Autodesk Inventor part; units mm, degrees
(part 2 of 2)
sketch "Sketch34" plane through (-87.5594, 7.4535, 25) normal (0, 1, 0) x (1, 0, 0)
  line L0 (67.0332, 20.1615) -> (71.3633, 20.1615)
  line L1 (71.3633, 20.1615) -> (73.5284, 16.4115)
  line L2 (73.5284, 16.4115) -> (71.3633, 12.6615)
  line L3 (71.3633, 12.6615) -> (67.0332, 12.6615)
  line L4 (67.0332, 12.6615) -> (64.8681, 16.4115)
  line L5 (64.8681, 16.4115) -> (67.0332, 20.1615)
  line L6 (76.0332, 14.75) -> (80.3633, 14.75)
  line L7 (80.3633, 14.75) -> (82.5284, 11)
  line L8 (82.5284, 11) -> (80.3633, 7.25)
  line L9 (80.3633, 7.25) -> (76.0332, 7.25)
  line L10 (76.0332, 7.25) -> (73.8681, 11)
  line L11 (73.8681, 11) -> (76.0332, 14.75)
  line L12 (67.0332, 30.9846) -> (71.3633, 30.9846)
  line L13 (71.3633, 30.9846) -> (73.5284, 27.2346)
  line L14 (73.5284, 27.2346) -> (71.3633, 23.4846)
  line L15 (71.3633, 23.4846) -> (67.0332, 23.4846)
  line L16 (67.0332, 23.4846) -> (64.8681, 27.2346)
  line L17 (64.8681, 27.2346) -> (67.0332, 30.9846)
  line L18 (76.0332, 25.5731) -> (80.3633, 25.5731)
  line L19 (80.3633, 25.5731) -> (82.5284, 21.8231)
  line L20 (82.5284, 21.8231) -> (80.3633, 18.0731)
  line L21 (80.3633, 18.0731) -> (76.0332, 18.0731)
  line L22 (76.0332, 18.0731) -> (73.8681, 21.8231)
  line L23 (73.8681, 21.8231) -> (76.0332, 25.5731)
  line L24 (55.8681, 21.8231) -> (58.0332, 25.5731)
  line L25 (58.0332, 25.5731) -> (62.3633, 25.5731)
  line L26 (62.3633, 25.5731) -> (64.5284, 21.8231)
  line L27 (58.0332, 18.0731) -> (55.8681, 21.8231)
  line L28 (64.5284, 21.8231) -> (62.3633, 18.0731)
  line L29 (62.3633, 18.0731) -> (58.0332, 18.0731)
  line L30 (58.0332, 14.75) -> (62.3633, 14.75)
  line L31 (55.8681, 11) -> (58.0332, 14.75)
  line L32 (58.0332, 7.25) -> (55.8681, 11)
  line L33 (62.3633, 14.75) -> (64.5284, 11)
  line L34 (62.3633, 7.25) -> (58.0332, 7.25)
  line L35 (64.5284, 11) -> (62.3633, 7.25)
  line L36 (49.0332, 20.1615) -> (53.3633, 20.1615)
  line L37 (53.3633, 20.1615) -> (55.5284, 16.4115)
  line L38 (55.5284, 16.4115) -> (53.3633, 12.6615)
  line L39 (53.3633, 12.6615) -> (49.0332, 12.6615)
  line L40 (49.0332, 12.6615) -> (46.8681, 16.4115)
  line L41 (46.8681, 16.4115) -> (49.0332, 20.1615)
  line L42 (53.3633, 23.4846) -> (49.0332, 23.4846)
  line L43 (55.5284, 27.2346) -> (53.3633, 23.4846)
  line L44 (53.3633, 30.9846) -> (55.5284, 27.2346)
  line L45 (49.0332, 23.4846) -> (46.8681, 27.2346)
  line L46 (49.0332, 30.9846) -> (53.3633, 30.9846)
  line L47 (46.8681, 27.2346) -> (49.0332, 30.9846)
  line L48 (53.3633, -1.1615) -> (55.5284, -4.9115)
  line L49 (55.5284, -4.9115) -> (53.3633, -8.6615)
  line L50 (53.3633, -8.6615) -> (49.0332, -8.6615)
  line L51 (49.0332, -8.6615) -> (46.8681, -4.9115)
  line L52 (49.0332, -1.1615) -> (53.3633, -1.1615)
  line L53 (46.8681, -4.9115) -> (49.0332, -1.1615)
  line L54 (67.0332, -1.1615) -> (71.3633, -1.1615)
  line L55 (71.3633, -1.1615) -> (73.5284, -4.9115)
  line L56 (80.3633, -3.25) -> (76.0332, -3.25)
  line L57 (76.0332, -3.25) -> (73.8681, 0.5)
  line L58 (82.5284, 0.5) -> (80.3633, -3.25)
  line L59 (80.3633, 4.25) -> (82.5284, 0.5)
  line L60 (76.0332, 4.25) -> (80.3633, 4.25)
  line L61 (73.8681, 0.5) -> (76.0332, 4.25)
  line L62 (71.3633, 2.1615) -> (67.0332, 2.1615)
  line L63 (73.5284, 5.9115) -> (71.3633, 2.1615)
  line L64 (67.0332, 9.6615) -> (71.3633, 9.6615)
  line L65 (71.3633, 9.6615) -> (73.5284, 5.9115)
  line L66 (58.0332, -3.25) -> (55.8681, 0.5)
  line L67 (55.8681, 0.5) -> (58.0332, 4.25)
  line L68 (58.0332, -6.5731) -> (62.3633, -6.5731)
  line L69 (62.3633, -3.25) -> (58.0332, -3.25)
  line L70 (58.0332, 4.25) -> (62.3633, 4.25)
  line L71 (62.3633, 4.25) -> (64.5284, 0.5)
  line L72 (64.5284, 0.5) -> (62.3633, -3.25)
  line L73 (64.8681, -4.9115) -> (67.0332, -1.1615)
  line L74 (67.0332, -8.6615) -> (64.8681, -4.9115)
  line L75 (67.0332, 2.1615) -> (64.8681, 5.9115)
  line L76 (64.8681, 5.9115) -> (67.0332, 9.6615)
  line L77 (73.5284, -4.9115) -> (71.3633, -8.6615)
  line L78 (71.3633, -8.6615) -> (67.0332, -8.6615)
  line L79 (76.0332, -6.5731) -> (80.3633, -6.5731)
  line L80 (73.8681, -10.3231) -> (76.0332, -6.5731)
  line L81 (76.0332, -14.0731) -> (73.8681, -10.3231)
  line L82 (80.3633, -6.5731) -> (82.5284, -10.3231)
  line L83 (80.3633, -14.0731) -> (76.0332, -14.0731)
  line L84 (82.5284, -10.3231) -> (80.3633, -14.0731)
  line L85 (55.8681, -10.3231) -> (58.0332, -6.5731)
  line L86 (62.3633, -6.5731) -> (64.5284, -10.3231)
  line L87 (62.3633, -14.0731) -> (58.0332, -14.0731)
  line L88 (64.5284, -10.3231) -> (62.3633, -14.0731)
  line L89 (58.0332, -14.0731) -> (55.8681, -10.3231)
  line L90 (53.3633, 2.1615) -> (49.0332, 2.1615)
  line L91 (55.5284, 5.9115) -> (53.3633, 2.1615)
  line L92 (49.0332, 2.1615) -> (46.8681, 5.9115)
  line L93 (46.8681, 5.9115) -> (49.0332, 9.6615)
  line L94 (53.3633, 9.6615) -> (55.5284, 5.9115)
  line L95 (49.0332, 9.6615) -> (53.3633, 9.6615)
  line L96 (51.1982, 27.2346) -> (51.1982, -4.9115) construction
  line L97 (31.0332, 9.6615) -> (28.8681, 5.9115)
  line L98 (28.8681, 16.4115) -> (31.0332, 12.6615)
  line L99 (35.3633, 9.6615) -> (31.0332, 9.6615)
  line L100 (31.0332, 12.6615) -> (35.3633, 12.6615)
  line L101 (35.3633, 12.6615) -> (37.5284, 16.4115)
  line L102 (37.5284, 5.9115) -> (35.3633, 9.6615)
  line L103 (37.8681, 11) -> (40.0332, 7.25)
  line L104 (40.0332, 14.75) -> (37.8681, 11)
  line L105 (26.3633, 7.25) -> (28.5284, 11)
  line L106 (28.5284, 11) -> (26.3633, 14.75)
  line L107 (26.3633, 14.75) -> (22.0332, 14.75)
  line L108 (22.0332, 7.25) -> (26.3633, 7.25)
  line L109 (22.0332, 14.75) -> (19.8681, 11)
  line L110 (19.8681, 11) -> (22.0332, 7.25)
  line L111 (26.3633, 4.25) -> (22.0332, 4.25)
  line L112 (22.0332, 4.25) -> (19.8681, 0.5)
  line L113 (28.8681, 5.9115) -> (31.0332, 2.1615)
  line L114 (28.5284, 0.5) -> (26.3633, 4.25)
  line L115 (37.8681, 21.8231) -> (40.0332, 18.0731)
  line L116 (44.3633, 25.5731) -> (40.0332, 25.5731)
  line L117 (40.0332, 18.0731) -> (44.3633, 18.0731)
  line L118 (46.5284, 21.8231) -> (44.3633, 25.5731)
  line L119 (44.3633, 18.0731) -> (46.5284, 21.8231)
  line L120 (44.3633, 14.75) -> (40.0332, 14.75)
  line L121 (46.5284, 11) -> (44.3633, 14.75)
  line L122 (44.3633, 7.25) -> (46.5284, 11)
  line L123 (19.8681, 0.5) -> (22.0332, -3.25)
  line L124 (22.0332, -3.25) -> (26.3633, -3.25)
  line L125 (31.0332, 2.1615) -> (35.3633, 2.1615)
  line L126 (26.3633, -3.25) -> (28.5284, 0.5)
  line L127 (35.3633, -1.1615) -> (31.0332, -1.1615)
  line L128 (31.0332, -1.1615) -> (28.8681, -4.9115)
  line L129 (35.3633, 20.1615) -> (31.0332, 20.1615)
  line L130 (31.0332, 20.1615) -> (28.8681, 16.4115)
  line L131 (37.5284, 16.4115) -> (35.3633, 20.1615)
  line L132 (35.3633, 30.9846) -> (31.0332, 30.9846)
  line L133 (31.0332, 30.9846) -> (28.8681, 27.2346)
  line L134 (28.8681, 27.2346) -> (31.0332, 23.4846)
  line L135 (31.0332, 23.4846) -> (35.3633, 23.4846)
  line L136 (35.3633, 23.4846) -> (37.5284, 27.2346)
  line L137 (40.0332, 25.5731) -> (37.8681, 21.8231)
  line L138 (37.5284, 27.2346) -> (35.3633, 30.9846)
  line L139 (26.3633, 18.0731) -> (28.5284, 21.8231)
  line L140 (28.5284, 21.8231) -> (26.3633, 25.5731)
  line L141 (22.0332, 18.0731) -> (26.3633, 18.0731)
  line L142 (26.3633, 25.5731) -> (22.0332, 25.5731)
  line L143 (22.0332, 25.5731) -> (19.8681, 21.8231)
  line L144 (19.8681, 21.8231) -> (22.0332, 18.0731)
  line L145 (40.0332, 7.25) -> (44.3633, 7.25)
  line L146 (35.3633, 2.1615) -> (37.5284, 5.9115)
  line L147 (37.5284, -4.9115) -> (35.3633, -1.1615)
  line L148 (40.0332, 4.25) -> (37.8681, 0.5)
  line L149 (37.8681, 0.5) -> (40.0332, -3.25)
  line L150 (44.3633, 4.25) -> (40.0332, 4.25)
  line L151 (40.0332, -3.25) -> (44.3633, -3.25)
  line L152 (46.5284, 0.5) -> (44.3633, 4.25)
  line L153 (44.3633, -3.25) -> (46.5284, 0.5)
  line L154 (31.0332, -8.6615) -> (35.3633, -8.6615)
  line L155 (28.8681, -4.9115) -> (31.0332, -8.6615)
  line L156 (28.5284, -10.3231) -> (26.3633, -6.5731)
  line L157 (26.3633, -14.0731) -> (28.5284, -10.3231)
  line L158 (22.0332, -14.0731) -> (26.3633, -14.0731)
  line L159 (26.3633, -6.5731) -> (22.0332, -6.5731)
  line L160 (19.8681, -10.3231) -> (22.0332, -14.0731)
  line L161 (22.0332, -6.5731) -> (19.8681, -10.3231)
  line L162 (35.3633, -8.6615) -> (37.5284, -4.9115)
  line L163 (37.8681, -10.3231) -> (40.0332, -14.0731)
  line L164 (40.0332, -6.5731) -> (37.8681, -10.3231)
  line L165 (44.3633, -6.5731) -> (40.0332, -6.5731)
  line L166 (46.5284, -10.3231) -> (44.3633, -6.5731)
  line L167 (44.3633, -14.0731) -> (46.5284, -10.3231)
  line L168 (40.0332, -14.0731) -> (44.3633, -14.0731)
  line L169 (24.1982, 21.8231) -> (24.1982, -10.3231) construction
  line L170 (10.8681, 16.4115) -> (13.0332, 20.1615)
  line L171 (13.0332, 12.6615) -> (10.8681, 16.4115)
  line L172 (10.8681, 5.9115) -> (13.0332, 9.6615)
  line L173 (17.3633, 9.6615) -> (19.5284, 5.9115)
  line L174 (19.5284, 16.4115) -> (17.3633, 12.6615)
  line L175 (19.5284, 5.9115) -> (17.3633, 2.1615)
  line L176 (17.3633, -1.1615) -> (19.5284, -4.9115)
  line L177 (19.5284, -4.9115) -> (17.3633, -8.6615)
  line L178 (13.0332, 23.4846) -> (10.8681, 27.2346)
  line L179 (10.8681, 27.2346) -> (13.0332, 30.9846)
  line L180 (13.0332, 20.1615) -> (17.3633, 20.1615)
  line L181 (17.3633, 23.4846) -> (13.0332, 23.4846)
  line L182 (13.0332, 30.9846) -> (17.3633, 30.9846)
  line L183 (13.0332, 9.6615) -> (17.3633, 9.6615)
  line L184 (17.3633, 12.6615) -> (13.0332, 12.6615)
  line L185 (17.3633, 20.1615) -> (19.5284, 16.4115)
  line L186 (13.0332, -8.6615) -> (10.8681, -4.9115)
  line L187 (13.0332, -1.1615) -> (17.3633, -1.1615)
  line L188 (17.3633, 2.1615) -> (13.0332, 2.1615)
  line L189 (17.3633, -8.6615) -> (13.0332, -8.6615)
  line L190 (13.0332, 2.1615) -> (10.8681, 5.9115)
  line L191 (10.8681, -4.9115) -> (13.0332, -1.1615)
  line L192 (17.3633, 30.9846) -> (19.5284, 27.2346)
  line L193 (19.5284, 27.2346) -> (17.3633, 23.4846)
  line L194 (1.8681, 0.5) -> (4.0332, 4.25)
  line L195 (4.0332, -3.25) -> (1.8681, 0.5)
  line L196 (1.8681, -10.3231) -> (4.0332, -6.5731)
  line L197 (4.0332, -6.5731) -> (8.3633, -6.5731)
  line L198 (8.3633, -14.0731) -> (4.0332, -14.0731)
  line L199 (8.3633, -6.5731) -> (10.5284, -10.3231)
  line L200 (10.5284, -10.3231) -> (8.3633, -14.0731)
  line L201 (4.0332, -14.0731) -> (1.8681, -10.3231)
  line L202 (8.3633, -3.25) -> (4.0332, -3.25)
  line L203 (8.3633, 4.25) -> (10.5284, 0.5)
  line L204 (10.5284, 0.5) -> (8.3633, -3.25)
  line L205 (4.0332, 4.25) -> (8.3633, 4.25)
  line L206 (8.3633, 25.5731) -> (10.5284, 21.8231)
  line L207 (10.5284, 21.8231) -> (8.3633, 18.0731)
  line L208 (4.0332, 25.5731) -> (8.3633, 25.5731)
  line L209 (1.8681, 21.8231) -> (4.0332, 25.5731)
  line L210 (4.0332, 18.0731) -> (1.8681, 21.8231)
  line L211 (8.3633, 18.0731) -> (4.0332, 18.0731)
  line L212 (8.3633, 7.25) -> (4.0332, 7.25)
  line L213 (10.5284, 11) -> (8.3633, 7.25)
  line L214 (4.0332, 7.25) -> (1.8681, 11)
  line L215 (1.8681, 11) -> (4.0332, 14.75)
  line L216 (8.3633, 14.75) -> (10.5284, 11)
  line L217 (4.0332, 14.75) -> (8.3633, 14.75)
  line L218 (15.1982, 27.2346) -> (69.1982, 27.2346) construction
  line L219 (10.5284, 32.6462) -> (8.3633, 36.3962)
  line L220 (4.0332, 36.3962) -> (1.8681, 32.6462)
  line L221 (1.8681, 32.6462) -> (4.0332, 28.8962)
  line L222 (4.0332, 28.8962) -> (8.3633, 28.8962)
  line L223 (8.3633, 28.8962) -> (10.5284, 32.6462)
  line L224 (8.3633, 36.3962) -> (4.0332, 36.3962)
  line L225 (26.3633, 36.3962) -> (28.5284, 32.6462)
  line L226 (28.5284, 32.6462) -> (26.3633, 28.8962)
  line L227 (22.0332, 36.3962) -> (26.3633, 36.3962)
  line L228 (19.8681, 32.6462) -> (22.0332, 36.3962)
  line L229 (26.3633, 28.8962) -> (22.0332, 28.8962)
  line L230 (22.0332, 28.8962) -> (19.8681, 32.6462)
  line L231 (24.1982, 32.6462) -> (24.1982, 64.7923) construction
  line L232 (37.8681, 32.6462) -> (40.0332, 36.3962)
  line L233 (40.0332, 28.8962) -> (37.8681, 32.6462)
  line L234 (44.3633, 28.8962) -> (40.0332, 28.8962)
  line L235 (40.0332, 36.3962) -> (44.3633, 36.3962)
  line L236 (44.3633, 36.3962) -> (46.5284, 32.6462)
  line L237 (46.5284, 32.6462) -> (44.3633, 28.8962)
  line L238 (64.5284, 32.6462) -> (62.3633, 36.3962)
  line L239 (58.0332, 28.8962) -> (62.3633, 28.8962)
  line L240 (62.3633, 28.8962) -> (64.5284, 32.6462)
  line L241 (55.8681, 32.6462) -> (58.0332, 28.8962)
  line L242 (58.0332, 36.3962) -> (55.8681, 32.6462)
  line L243 (76.0332, 36.3962) -> (73.8681, 32.6462)
  line L244 (73.8681, 32.6462) -> (76.0332, 28.8962)
  line L245 (80.3633, 36.3962) -> (76.0332, 36.3962)
  line L246 (76.0332, 28.8962) -> (80.3633, 28.8962)
  line L247 (80.3633, 28.8962) -> (82.5284, 32.6462)
  line L248 (82.5284, 32.6462) -> (80.3633, 36.3962)
  line L249 (62.3633, 36.3962) -> (58.0332, 36.3962)
  line L250 (6.1982, 11) -> (78.1982, 11) construction
  circle A0 centre (-86.043, -4) radius 2.45 construction
  circle A1 centre (-86.043, -72.2) radius 2.45 construction
  line L251 (-86.043, -4) -> (-86.043, -72.2) construction
  line L252 (-86.043, -4) -> (-4.4209, -4) construction
  line L253 (42.1982, 32.6462) -> (42.1982, -10.3231) construction
  line L254 (0, 0) -> (84.3965, 0) projected
  line L255 (-10, 22) -> (-10, 0) projected
  point P0 (87.5594, 25)
  point P1 (69.1982, 16.4115)
  point P2 (78.1982, 21.8231)
  point P3 (60.1982, 11)
  point P4 (60.1982, 21.8231)
  point P5 (51.1982, 16.4115)
  point P6 (78.1982, 0.5)
  point P7 (69.1982, 5.9115)
  point P8 (60.1982, 0.5)
  point P9 (69.1982, -4.9115)
  point P10 (78.1982, -10.3231)
  point P11 (60.1982, -10.3231)
  point P12 (51.1982, 5.9115)
  point P13 (33.1982, 5.9115)
  point P14 (33.1982, 16.4115)
  point P15 (24.1982, 11)
  point P16 (24.1982, 0.5)
  point P17 (42.1982, 21.8231)
  point P18 (42.1982, 11)
  point P19 (33.1982, 27.2346)
  point P20 (42.1982, 0.5)
  point P21 (33.1982, -4.9115)
  point P22 (15.1982, 5.9115)
  point P23 (15.1982, 16.4115)
  point P24 (15.1982, -4.9115)
  point P25 (6.1982, -10.3231)
  point P26 (6.1982, 0.5)
  point P27 (6.1982, 21.8231)
  point P28 (6.1982, 32.6462)
  point P29 (60.1982, 32.6462)
  point P30 (78.1982, 32.6462)
  point P31 (-86.043, -38.1)
  point P32 (-45.232, -4)
  point P33 (42.1982, -6.5731)
  point P34 (42.1982, 0)
  point P35 (-10, 11)
  point P36 (42.1982, 11)
  dimension "d219" = 7.5
  dimension "d220" = 7.5
  dimension "d221" = 3
  dimension "d222" = 7.5
  dimension "d223" = 7.5
  dimension "d224" = 3
  dimension "d225" = 3
  dimension "d226" = 18
  dimension "d227" = 3
  dimension "d228" = 3
  dimension "d229" = 7.5
  dimension "d230" = 7.5
  dimension "d231" = 3
  dimension "d232" = 7.5
  dimension "d233" = 7.5
  dimension "d234" = 3
  dimension "d235" = 3
  dimension "d236" = 18
  dimension "d237" = 3
  dimension "d238" = 3
  dimension "d239" = 3
  constraints: 508 end point, 176 symmetric about line, 6 midpoint, 5 vertical alignment, 3 horizontal, 2 centre point, 2 collinear, 2 vertical, 1 horizontal alignment, 206 other
  measures "d219" distance between parallel lines of L0 L3
  measures "d220" distance between parallel lines of L6 L9
  measures "d221" distance between parallel lines of L2 L11
  measures "d222" distance between parallel lines of L12 L15
  measures "d223" distance between parallel lines of L18 L21
  measures "d224" distance between parallel lines of L14 L23
  measures "d225" distance between parallel lines of L22 L1
  measures "d226" distance of L250.end point (60.198, 11)
  measures "d227" distance between parallel lines of L5 L28
  measures "d228" distance between parallel lines of L4 L33
  measures "d229" distance between parallel lines of L54 L78
  measures "d230" distance between parallel lines of L79 L83
  measures "d231" distance between parallel lines of L77 L80
  measures "d232" distance between parallel lines of L64 L62
  measures "d233" distance between parallel lines of L60 L56
  measures "d234" distance between parallel lines of L63 L61
  measures "d235" distance between parallel lines of L57 L55
  measures "d236" distance of point (78.198, -10.323) point (60.198, -10.323)
  measures "d237" distance between parallel lines of L73 L72
  measures "d238" distance between parallel lines of L74 L86
  measures "d239" distance of L59.start L8.end
extrude "Extrusion31" cut sketch "Sketch34" against normal blind 10 contours L0 L1 L2 L3 L4 L5 | L6 L7 L8 L9 L10 L11 | L30 L33 L35 L34 L32 L31 | L36 L37 L38 L39 L40 L41 | L62 L75 L76 L64 L65 L63 | L90 L92 L93 L95 L94 L91 | L99 L102 L146 L125 L113 L97 | L130 L129 L131 L101 L100 L98 | L104 L120 L121 L122 L145 L103 | L108 L110 L109 L107 L106 L105 | L170 L180 L185 L174 L184 L171 | L172 L183 L173 L175 L188 L190 | L212 L214 L215 L217 L216 L213
sketch "Sketch35" plane through (-87.5594, -167.9139, 25) normal (0, -1, 0) x (1, 0, 0)
  point P0 (87.5594, -25)
extrude "Extrusion32" cut sketch "Sketch34" against normal blind 10 from surface at -171.3673 contours L0 L1 L2 L3 L4 L5 | L6 L7 L8 L9 L10 L11 | L30 L33 L35 L34 L32 L31 | L36 L37 L38 L39 L40 L41 | L62 L75 L76 L64 L65 L63 | L90 L92 L93 L95 L94 L91 | L99 L102 L146 L125 L113 L97 | L130 L129 L131 L101 L100 L98 | L104 L120 L121 L122 L145 L103 | L108 L110 L109 L107 L106 L105 | L170 L180 L185 L174 L184 L171 | L172 L183 L173 L175 L188 L190 | L212 L214 L215 L217 L216 L213
body "Solid2"
